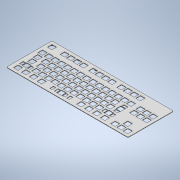
# Autodesk Inventor part: Plate
Saved by Autodesk Inventor 2022 (Build 260153000, 153)
## iProperties
Created: 2021-09-06
Part Number: Plate
Material: 一般
Document SubType Name: Modeling
Designer: shiok
Density: 1 g/cm^3
Appearance: 既定
Author: shiok
## iProperties of the stored document Plate_3D プリント.ipt
Created: 2021-09-06
Part Number: Plate_3D プリント
Material: 一般
Document SubType Name: Modeling
Designer: shiok
Density: 1 g/cm^3
Appearance: 既定
Author: shiok
Autodesk Inventor part; units mm, degrees
(part 1 of 3)
ref_plane "YZ Plane" through (0, 0, 0) normal (1, 0, 0) x (0, 1, 0)
ref_plane "XZ Plane" through (0, 0, 0) normal (0, 1, 0) x (-1, 0, 0)
ref_plane "XY Plane" through (0, 0, 0) normal (0, 0, 1) x (1, 0, 0)
sketch "スケッチ1" plane through (0, 0, 0) normal (0, 1, 0) x (-1, 0, 0)
  line L0 (180.1975, -68.58) -> (-180.1975, -68.58)
  line L1 (-183.1975, -65.58) -> (-183.1975, 65.58)
  line L2 (-180.1975, 68.58) -> (180.1975, 68.58)
  line L3 (183.1975, 65.58) -> (183.1975, -65.58)
  line L4 (183.1975, 68.58) -> (-183.1975, -68.58) construction
  line L5 (183.1975, -68.58) -> (-183.1975, 68.58) construction
  arc A0 (180.1975, -68.58) -> (183.1975, -65.58) centre (180.1975, -65.58) ccw
  arc A1 (183.1975, 65.58) -> (180.1975, 68.58) centre (180.1975, 65.58) ccw
  arc A2 (-180.1975, 68.58) -> (-183.1975, 65.58) centre (-180.1975, 65.58) ccw
  arc A3 (-183.1975, -65.58) -> (-180.1975, -68.58) centre (-180.1975, -65.58) ccw
  line L6 (135.3312, -59.0677) -> (121.8438, -59.0677)
  line L7 (121.5898, -58.8137) -> (121.5898, -45.3263)
  line L8 (121.8438, -45.0723) -> (135.3312, -45.0723)
  line L9 (135.5852, -45.3263) -> (135.5852, -58.8137)
  line L10 (135.5852, -59.0677) -> (121.5898, -45.0723) construction
  line L11 (121.5898, -59.0677) -> (135.5852, -45.0723) construction
  arc A4 (135.3312, -59.0677) -> (135.5852, -58.8137) centre (135.3312, -58.8137) ccw
  arc A5 (121.5898, -58.8137) -> (121.8438, -59.0677) centre (121.8438, -58.8137) ccw
  arc A6 (121.8438, -45.0723) -> (121.5898, -45.3263) centre (121.8438, -45.3263) ccw
  arc A7 (135.5852, -45.3263) -> (135.3312, -45.0723) centre (135.3312, -45.3263) ccw
  line L12 (116.5352, -45.3263) -> (116.5352, -58.8137)
  arc A8 (116.5352, -45.3263) -> (116.2812, -45.0723) centre (116.2812, -45.3263) ccw
  arc A9 (116.2812, -59.0677) -> (116.5352, -58.8137) centre (116.2812, -58.8137) ccw
  line L13 (116.2812, -59.0677) -> (102.7938, -59.0677)
  line L14 (102.7938, -45.0723) -> (116.2812, -45.0723)
  line L15 (116.5352, -59.0677) -> (102.5398, -45.0723) construction
  line L16 (102.5398, -59.0677) -> (116.5352, -45.0723) construction
  arc A10 (102.7938, -45.0723) -> (102.5398, -45.3263) centre (102.7938, -45.3263) ccw
  line L17 (102.5398, -58.8137) -> (102.5398, -45.3263)
  arc A11 (102.5398, -58.8137) -> (102.7938, -59.0677) centre (102.7938, -58.8137) ccw
  line L18 (97.4852, -45.3263) -> (97.4852, -58.8137)
  arc A12 (97.4852, -45.3263) -> (97.2312, -45.0723) centre (97.2312, -45.3263) ccw
  arc A13 (97.2312, -59.0677) -> (97.4852, -58.8137) centre (97.2312, -58.8137) ccw
  line L19 (97.2312, -59.0677) -> (83.7438, -59.0677)
  line L20 (83.7438, -45.0723) -> (97.2312, -45.0723)
  line L21 (97.4852, -59.0677) -> (83.4898, -45.0723) construction
  line L22 (83.4898, -59.0677) -> (97.4852, -45.0723) construction
  arc A14 (83.7438, -45.0723) -> (83.4898, -45.3263) centre (83.7438, -45.3263) ccw
  line L23 (83.4898, -58.8137) -> (83.4898, -45.3263)
  arc A15 (83.4898, -58.8137) -> (83.7438, -59.0677) centre (83.7438, -58.8137) ccw
  line L24 (78.4352, -45.3263) -> (78.4352, -58.8137)
  arc A16 (78.4352, -45.3263) -> (78.1812, -45.0723) centre (78.1812, -45.3263) ccw
  arc A17 (78.1812, -59.0677) -> (78.4352, -58.8137) centre (78.1812, -58.8137) ccw
  line L25 (78.1812, -59.0677) -> (64.6938, -59.0677)
  line L26 (64.6938, -45.0723) -> (78.1812, -45.0723)
  line L27 (78.4352, -59.0677) -> (64.4398, -45.0723) construction
  line L28 (64.4398, -59.0677) -> (78.4352, -45.0723) construction
  arc A18 (64.6938, -45.0723) -> (64.4398, -45.3263) centre (64.6938, -45.3263) ccw
  line L29 (64.4398, -58.8137) -> (64.4398, -45.3263)
  arc A19 (64.4398, -58.8137) -> (64.6938, -59.0677) centre (64.6938, -58.8137) ccw
  line L30 (36.1188, -45.0723) -> (49.6062, -45.0723)
  line L31 (35.8648, -58.8137) -> (35.8648, -45.3263)
  line L32 (49.8602, -45.3263) -> (49.8602, -58.8137)
  line L33 (49.8602, -59.0677) -> (35.8648, -45.0723) construction
  line L34 (35.8648, -59.0677) -> (49.8602, -45.0723) construction
  arc A20 (49.6062, -59.0677) -> (49.8602, -58.8137) centre (49.6062, -58.8137) ccw
  arc A21 (35.8648, -58.8137) -> (36.1188, -59.0677) centre (36.1188, -58.8137) ccw
  line L35 (30.8102, -45.3263) -> (30.8102, -58.8137)
  line L36 (49.6062, -59.0677) -> (36.1188, -59.0677)
  arc A22 (49.8602, -45.3263) -> (49.6062, -45.0723) centre (49.6062, -45.3263) ccw
  arc A23 (36.1188, -45.0723) -> (35.8648, -45.3263) centre (36.1188, -45.3263) ccw
  arc A24 (30.8102, -45.3263) -> (30.5562, -45.0723) centre (30.5562, -45.3263) ccw
  arc A25 (30.5562, -59.0677) -> (30.8102, -58.8137) centre (30.5562, -58.8137) ccw
  line L37 (17.0688, -45.0723) -> (30.5562, -45.0723)
  line L38 (30.5562, -59.0677) -> (17.0688, -59.0677)
  line L39 (30.8102, -59.0677) -> (16.8148, -45.0723) construction
  line L40 (16.8148, -59.0677) -> (30.8102, -45.0723) construction
  arc A26 (17.0688, -45.0723) -> (16.8148, -45.3263) centre (17.0688, -45.3263) ccw
  line L41 (16.8148, -58.8137) -> (16.8148, -45.3263)
  arc A27 (16.8148, -58.8137) -> (17.0688, -59.0677) centre (17.0688, -58.8137) ccw
  line L42 (11.7602, -45.3263) -> (11.7602, -58.8137)
  arc A28 (11.7602, -45.3263) -> (11.5062, -45.0723) centre (11.5062, -45.3263) ccw
  arc A29 (11.5062, -59.0677) -> (11.7602, -58.8137) centre (11.5062, -58.8137) ccw
  line L43 (11.5062, -59.0677) -> (-1.9812, -59.0677)
  line L44 (-1.9812, -45.0723) -> (11.5062, -45.0723)
  line L45 (11.7602, -59.0677) -> (-2.2352, -45.0723) construction
  line L46 (-2.2352, -59.0677) -> (11.7602, -45.0723) construction
  arc A30 (-2.2352, -58.8137) -> (-1.9812, -59.0677) centre (-1.9812, -58.8137) ccw
  arc A31 (-7.5438, -59.0677) -> (-7.2898, -58.8137) centre (-7.5438, -58.8137) ccw
  arc A32 (-1.9812, -45.0723) -> (-2.2352, -45.3263) centre (-1.9812, -45.3263) ccw
  line L47 (-2.2352, -58.8137) -> (-2.2352, -45.3263)
  line L48 (-7.2898, -45.3263) -> (-7.2898, -58.8137)
  line L49 (-7.5438, -59.0677) -> (-21.0312, -59.0677)
  arc A33 (-21.2852, -58.8137) -> (-21.0312, -59.0677) centre (-21.0312, -58.8137) ccw
  arc A34 (-7.2898, -45.3263) -> (-7.5438, -45.0723) centre (-7.5438, -45.3263) ccw
  line L50 (-21.0312, -45.0723) -> (-7.5438, -45.0723)
  line L51 (-21.2852, -58.8137) -> (-21.2852, -45.3263)
  line L52 (-21.2852, -59.0677) -> (-7.2898, -45.0723) construction
  arc A35 (-21.0312, -45.0723) -> (-21.2852, -45.3263) centre (-21.0312, -45.3263) ccw
  line L53 (-7.2898, -59.0677) -> (-21.2852, -45.0723) construction
  line L54 (-49.6062, -45.0723) -> (-36.1188, -45.0723)
  line L55 (-49.8602, -58.8137) -> (-49.8602, -45.3263)
  line L56 (-35.8648, -45.3263) -> (-35.8648, -58.8137)
  line L57 (-35.8648, -59.0677) -> (-49.8602, -45.0723) construction
  line L58 (-49.8602, -59.0677) -> (-35.8648, -45.0723) construction
  arc A36 (-36.1188, -59.0677) -> (-35.8648, -58.8137) centre (-36.1188, -58.8137) ccw
  arc A37 (-49.8602, -58.8137) -> (-49.6062, -59.0677) centre (-49.6062, -58.8137) ccw
  line L59 (-54.9148, -45.3263) -> (-54.9148, -58.8137)
  line L60 (-36.1188, -59.0677) -> (-49.6062, -59.0677)
  arc A38 (-35.8648, -45.3263) -> (-36.1188, -45.0723) centre (-36.1188, -45.3263) ccw
  arc A39 (-49.6062, -45.0723) -> (-49.8602, -45.3263) centre (-49.6062, -45.3263) ccw
  arc A40 (-54.9148, -45.3263) -> (-55.1688, -45.0723) centre (-55.1688, -45.3263) ccw
  arc A41 (-55.1688, -59.0677) -> (-54.9148, -58.8137) centre (-55.1688, -58.8137) ccw
  line L61 (-68.6562, -45.0723) -> (-55.1688, -45.0723)
  line L62 (-55.1688, -59.0677) -> (-68.6562, -59.0677)
  line L63 (-54.9148, -59.0677) -> (-68.9102, -45.0723) construction
  line L64 (-68.9102, -59.0677) -> (-54.9148, -45.0723) construction
  arc A42 (-68.6562, -45.0723) -> (-68.9102, -45.3263) centre (-68.6562, -45.3263) ccw
  line L65 (-68.9102, -58.8137) -> (-68.9102, -45.3263)
  arc A43 (-68.9102, -58.8137) -> (-68.6562, -59.0677) centre (-68.6562, -58.8137) ccw
  line L66 (-73.9648, -45.3263) -> (-73.9648, -58.8137)
  arc A44 (-73.9648, -45.3263) -> (-74.2188, -45.0723) centre (-74.2188, -45.3263) ccw
  arc A45 (-74.2188, -59.0677) -> (-73.9648, -58.8137) centre (-74.2188, -58.8137) ccw
  line L67 (-74.2188, -59.0677) -> (-87.7062, -59.0677)
  line L68 (-87.7062, -45.0723) -> (-74.2188, -45.0723)
  line L69 (-73.9648, -59.0677) -> (-87.9602, -45.0723) construction
  line L70 (-87.9602, -59.0677) -> (-73.9648, -45.0723) construction
  arc A46 (-87.9602, -58.8137) -> (-87.7062, -59.0677) centre (-87.7062, -58.8137) ccw
  arc A47 (-93.2688, -59.0677) -> (-93.0148, -58.8137) centre (-93.2688, -58.8137) ccw
  arc A48 (-87.7062, -45.0723) -> (-87.9602, -45.3263) centre (-87.7062, -45.3263) ccw
  line L71 (-87.9602, -58.8137) -> (-87.9602, -45.3263)
  line L72 (-93.0148, -45.3263) -> (-93.0148, -58.8137)
  line L73 (-93.2688, -59.0677) -> (-106.7562, -59.0677)
  arc A49 (-107.0102, -58.8137) -> (-106.7562, -59.0677) centre (-106.7562, -58.8137) ccw
  arc A50 (-93.0148, -45.3263) -> (-93.2688, -45.0723) centre (-93.2688, -45.3263) ccw
  line L74 (-106.7562, -45.0723) -> (-93.2688, -45.0723)
  line L75 (-107.0102, -58.8137) -> (-107.0102, -45.3263)
  line L76 (-107.0102, -59.0677) -> (-93.0148, -45.0723) construction
  arc A51 (-106.7562, -45.0723) -> (-107.0102, -45.3263) centre (-106.7562, -45.3263) ccw
  line L77 (-93.0148, -59.0677) -> (-107.0102, -45.0723) construction
  line L78 (128.5875, -68.58) -> (128.5875, -52.07) construction
  line L79 (128.5875, -52.07) -> (183.1975, -52.07) construction
  line L80 (173.4312, -30.4927) -> (159.9438, -30.4927)
  line L81 (159.6898, -30.2387) -> (159.6898, -16.7513)
  line L82 (159.9438, -16.4973) -> (173.4312, -16.4973)
  line L83 (173.6852, -16.7513) -> (173.6852, -30.2387)
  line L84 (173.6852, -30.4927) -> (159.6898, -16.4973) construction
  line L85 (159.6898, -30.4927) -> (173.6852, -16.4973) construction
  arc A52 (173.4312, -30.4927) -> (173.6852, -30.2387) centre (173.4312, -30.2387) ccw
  arc A53 (159.6898, -30.2387) -> (159.9438, -30.4927) centre (159.9438, -30.2387) ccw
  arc A54 (159.9438, -16.4973) -> (159.6898, -16.7513) centre (159.9438, -16.7513) ccw
  arc A55 (173.6852, -16.7513) -> (173.4312, -16.4973) centre (173.4312, -16.7513) ccw
  line L86 (76.6706, -116.022) -> (63.1832, -116.022)
  line L87 (62.9292, -115.768) -> (62.9292, -102.2806)
  line L88 (63.1832, -102.0266) -> (76.6706, -102.0266)
  line L89 (76.9246, -102.2806) -> (76.9246, -115.768)
  line L90 (76.9246, -116.022) -> (62.9292, -102.0266) construction
  line L91 (62.9292, -116.022) -> (76.9246, -102.0266) construction
  arc A56 (76.6706, -116.022) -> (76.9246, -115.768) centre (76.6706, -115.768) ccw
  arc A57 (62.9292, -115.768) -> (63.1832, -116.022) centre (63.1832, -115.768) ccw
  arc A58 (63.1832, -102.0266) -> (62.9292, -102.2806) centre (63.1832, -102.2806) ccw
  arc A59 (76.9246, -102.2806) -> (76.6706, -102.0266) centre (76.6706, -102.2806) ccw
  line L92 (173.4312, -59.0677) -> (159.9438, -59.0677)
  line L93 (159.6898, -58.8137) -> (159.6898, -45.3263)
  line L94 (159.9438, -45.0723) -> (173.4312, -45.0723)
  line L95 (173.6852, -45.3263) -> (173.6852, -58.8137)
  line L96 (173.6852, -59.0677) -> (159.6898, -45.0723) construction
  line L97 (159.6898, -59.0677) -> (173.6852, -45.0723) construction
  arc A60 (173.4312, -59.0677) -> (173.6852, -58.8137) centre (173.4312, -58.8137) ccw
  arc A61 (159.6898, -58.8137) -> (159.9438, -59.0677) centre (159.9438, -58.8137) ccw
  arc A62 (159.9438, -45.0723) -> (159.6898, -45.3263) centre (159.9438, -45.3263) ccw
  arc A63 (173.6852, -45.3263) -> (173.4312, -45.0723) centre (173.4312, -45.3263) ccw
  arc A64 (135.5852, 40.3987) -> (135.3312, 40.6527) centre (135.3312, 40.3987) ccw
  line L98 (135.5852, 40.3987) -> (135.5852, 26.9113)
  arc A65 (135.3312, 26.6573) -> (135.5852, 26.9113) centre (135.3312, 26.9113) ccw
  line L99 (121.8438, 40.6527) -> (135.3312, 40.6527)
  line L100 (135.3312, 26.6573) -> (121.8438, 26.6573)
  line L101 (135.5852, 26.6573) -> (121.5898, 40.6527) construction
  line L102 (121.5898, 26.6573) -> (135.5852, 40.6527) construction
  arc A66 (121.5898, 26.9113) -> (121.8438, 26.6573) centre (121.8438, 26.9113) ccw
  line L103 (121.5898, 26.9113) -> (121.5898, 40.3987)
  arc A67 (121.8438, 40.6527) -> (121.5898, 40.3987) centre (121.8438, 40.3987) ccw
  line L104 (154.3812, -30.4927) -> (140.8938, -30.4927)
  line L105 (140.6398, -30.2387) -> (140.6398, -16.7513)
  line L106 (140.8938, -16.4973) -> (154.3812, -16.4973)
  line L107 (154.6352, -16.7513) -> (154.6352, -30.2387)
  line L108 (154.6352, -30.4927) -> (140.6398, -16.4973) construction
  line L109 (140.6398, -30.4927) -> (154.6352, -16.4973) construction
  arc A68 (154.3812, -30.4927) -> (154.6352, -30.2387) centre (154.3812, -30.2387) ccw
  arc A69 (140.6398, -30.2387) -> (140.8938, -30.4927) centre (140.8938, -30.2387) ccw
  arc A70 (140.8938, -16.4973) -> (140.6398, -16.7513) centre (140.8938, -16.7513) ccw
  arc A71 (154.6352, -16.7513) -> (154.3812, -16.4973) centre (154.3812, -16.7513) ccw
  line L110 (135.3312, -30.4927) -> (121.8438, -30.4927)
  line L111 (121.5898, -30.2387) -> (121.5898, -16.7513)
  line L112 (121.8438, -16.4973) -> (135.3312, -16.4973)
  line L113 (135.5852, -16.7513) -> (135.5852, -30.2387)
  line L114 (135.5852, -30.4927) -> (121.5898, -16.4973) construction
  line L115 (121.5898, -30.4927) -> (135.5852, -16.4973) construction
  arc A72 (135.3312, -30.4927) -> (135.5852, -30.2387) centre (135.3312, -30.2387) ccw
  arc A73 (121.5898, -30.2387) -> (121.8438, -30.4927) centre (121.8438, -30.2387) ccw
  arc A74 (121.8438, -16.4973) -> (121.5898, -16.7513) centre (121.8438, -16.7513) ccw
  arc A75 (135.5852, -16.7513) -> (135.3312, -16.4973) centre (135.3312, -16.7513) ccw
  line L116 (116.2812, -30.4927) -> (102.7938, -30.4927)
  line L117 (102.5398, -30.2387) -> (102.5398, -16.7513)
  line L118 (102.7938, -16.4973) -> (116.2812, -16.4973)
  line L119 (116.5352, -16.7513) -> (116.5352, -30.2387)
  line L120 (116.5352, -30.4927) -> (102.5398, -16.4973) construction
  line L121 (102.5398, -30.4927) -> (116.5352, -16.4973) construction
  arc A76 (116.2812, -30.4927) -> (116.5352, -30.2387) centre (116.2812, -30.2387) ccw
  arc A77 (102.5398, -30.2387) -> (102.7938, -30.4927) centre (102.7938, -30.2387) ccw
  arc A78 (102.7938, -16.4973) -> (102.5398, -16.7513) centre (102.7938, -16.7513) ccw
  arc A79 (116.5352, -16.7513) -> (116.2812, -16.4973) centre (116.2812, -16.7513) ccw
  line L122 (97.2312, -30.4927) -> (83.7438, -30.4927)
  line L123 (83.4898, -30.2387) -> (83.4898, -16.7513)
  line L124 (83.7438, -16.4973) -> (97.2312, -16.4973)
  line L125 (97.4852, -16.7513) -> (97.4852, -30.2387)
  line L126 (97.4852, -30.4927) -> (83.4898, -16.4973) construction
  line L127 (83.4898, -30.4927) -> (97.4852, -16.4973) construction
  arc A80 (97.2312, -30.4927) -> (97.4852, -30.2387) centre (97.2312, -30.2387) ccw
  arc A81 (83.4898, -30.2387) -> (83.7438, -30.4927) centre (83.7438, -30.2387) ccw
  arc A82 (83.7438, -16.4973) -> (83.4898, -16.7513) centre (83.7438, -16.7513) ccw
  arc A83 (97.4852, -16.7513) -> (97.2312, -16.4973) centre (97.2312, -16.7513) ccw
  line L128 (78.1812, -30.4927) -> (64.6938, -30.4927)
  line L129 (64.4398, -30.2387) -> (64.4398, -16.7513)
  line L130 (64.6938, -16.4973) -> (78.1812, -16.4973)
  line L131 (78.4352, -16.7513) -> (78.4352, -30.2387)
  line L132 (78.4352, -30.4927) -> (64.4398, -16.4973) construction
  line L133 (64.4398, -30.4927) -> (78.4352, -16.4973) construction
  arc A84 (78.1812, -30.4927) -> (78.4352, -30.2387) centre (78.1812, -30.2387) ccw
  arc A85 (64.4398, -30.2387) -> (64.6938, -30.4927) centre (64.6938, -30.2387) ccw
  arc A86 (64.6938, -16.4973) -> (64.4398, -16.7513) centre (64.6938, -16.7513) ccw
  arc A87 (78.4352, -16.7513) -> (78.1812, -16.4973) centre (78.1812, -16.7513) ccw
  line L134 (59.1312, -30.4927) -> (45.6438, -30.4927)
  line L135 (45.3898, -30.2387) -> (45.3898, -16.7513)
  line L136 (45.6438, -16.4973) -> (59.1312, -16.4973)
  line L137 (59.3852, -16.7513) -> (59.3852, -30.2387)
  line L138 (59.3852, -30.4927) -> (45.3898, -16.4973) construction
  line L139 (45.3898, -30.4927) -> (59.3852, -16.4973) construction
  arc A88 (59.1312, -30.4927) -> (59.3852, -30.2387) centre (59.1312, -30.2387) ccw
  arc A89 (45.3898, -30.2387) -> (45.6438, -30.4927) centre (45.6438, -30.2387) ccw
  arc A90 (45.6438, -16.4973) -> (45.3898, -16.7513) centre (45.6438, -16.7513) ccw
  arc A91 (59.3852, -16.7513) -> (59.1312, -16.4973) centre (59.1312, -16.7513) ccw
  line L140 (40.0812, -30.4927) -> (26.5938, -30.4927)
  line L141 (26.3398, -30.2387) -> (26.3398, -16.7513)
  line L142 (26.5938, -16.4973) -> (40.0812, -16.4973)
  line L143 (40.3352, -16.7513) -> (40.3352, -30.2387)
  line L144 (40.3352, -30.4927) -> (26.3398, -16.4973) construction
  line L145 (26.3398, -30.4927) -> (40.3352, -16.4973) construction
  arc A92 (40.0812, -30.4927) -> (40.3352, -30.2387) centre (40.0812, -30.2387) ccw
  arc A93 (26.3398, -30.2387) -> (26.5938, -30.4927) centre (26.5938, -30.2387) ccw
  arc A94 (26.5938, -16.4973) -> (26.3398, -16.7513) centre (26.5938, -16.7513) ccw
  arc A95 (40.3352, -16.7513) -> (40.0812, -16.4973) centre (40.0812, -16.7513) ccw
  line L146 (21.0312, -30.4927) -> (7.5438, -30.4927)
  line L147 (7.2898, -30.2387) -> (7.2898, -16.7513)
  line L148 (7.5438, -16.4973) -> (21.0312, -16.4973)
  line L149 (21.2852, -16.7513) -> (21.2852, -30.2387)
  line L150 (21.2852, -30.4927) -> (7.2898, -16.4973) construction
  line L151 (7.2898, -30.4927) -> (21.2852, -16.4973) construction
  arc A96 (21.0312, -30.4927) -> (21.2852, -30.2387) centre (21.0312, -30.2387) ccw
  arc A97 (7.2898, -30.2387) -> (7.5438, -30.4927) centre (7.5438, -30.2387) ccw
  arc A98 (7.5438, -16.4973) -> (7.2898, -16.7513) centre (7.5438, -16.7513) ccw
  arc A99 (21.2852, -16.7513) -> (21.0312, -16.4973) centre (21.0312, -16.7513) ccw
  line L152 (1.9812, -30.4927) -> (-11.5062, -30.4927)
  line L153 (-11.7602, -30.2387) -> (-11.7602, -16.7513)
  line L154 (-11.5062, -16.4973) -> (1.9812, -16.4973)
  line L155 (2.2352, -16.7513) -> (2.2352, -30.2387)
  line L156 (2.2352, -30.4927) -> (-11.7602, -16.4973) construction
  line L157 (-11.7602, -30.4927) -> (2.2352, -16.4973) construction
  arc A100 (1.9812, -30.4927) -> (2.2352, -30.2387) centre (1.9812, -30.2387) ccw
  arc A101 (-11.7602, -30.2387) -> (-11.5062, -30.4927) centre (-11.5062, -30.2387) ccw
  arc A102 (-11.5062, -16.4973) -> (-11.7602, -16.7513) centre (-11.5062, -16.7513) ccw
  arc A103 (2.2352, -16.7513) -> (1.9812, -16.4973) centre (1.9812, -16.7513) ccw
  line L158 (-17.0688, -30.4927) -> (-30.5562, -30.4927)
  line L159 (-30.8102, -30.2387) -> (-30.8102, -16.7513)
  line L160 (-30.5562, -16.4973) -> (-17.0688, -16.4973)
  line L161 (-16.8148, -16.7513) -> (-16.8148, -30.2387)
  line L162 (-16.8148, -30.4927) -> (-30.8102, -16.4973) construction
  line L163 (-30.8102, -30.4927) -> (-16.8148, -16.4973) construction
  arc A104 (-17.0688, -30.4927) -> (-16.8148, -30.2387) centre (-17.0688, -30.2387) ccw
  arc A105 (-30.8102, -30.2387) -> (-30.5562, -30.4927) centre (-30.5562, -30.2387) ccw
  arc A106 (-30.5562, -16.4973) -> (-30.8102, -16.7513) centre (-30.5562, -16.7513) ccw
  arc A107 (-16.8148, -16.7513) -> (-17.0688, -16.4973) centre (-17.0688, -16.7513) ccw
  line L164 (-36.1188, -30.4927) -> (-49.6062, -30.4927)
  line L165 (-49.8602, -30.2387) -> (-49.8602, -16.7513)
  line L166 (-49.6062, -16.4973) -> (-36.1188, -16.4973)
  line L167 (-35.8648, -16.7513) -> (-35.8648, -30.2387)
  line L168 (-35.8648, -30.4927) -> (-49.8602, -16.4973) construction
  line L169 (-49.8602, -30.4927) -> (-35.8648, -16.4973) construction
  arc A108 (-36.1188, -30.4927) -> (-35.8648, -30.2387) centre (-36.1188, -30.2387) ccw
  arc A109 (-49.8602, -30.2387) -> (-49.6062, -30.4927) centre (-49.6062, -30.2387) ccw
  arc A110 (-49.6062, -16.4973) -> (-49.8602, -16.7513) centre (-49.6062, -16.7513) ccw
  arc A111 (-35.8648, -16.7513) -> (-36.1188, -16.4973) centre (-36.1188, -16.7513) ccw
  line L170 (-55.1688, -30.4927) -> (-68.6562, -30.4927)
  line L171 (-68.9102, -30.2387) -> (-68.9102, -16.7513)
  line L172 (-68.6562, -16.4973) -> (-55.1688, -16.4973)
  line L173 (-54.9148, -16.7513) -> (-54.9148, -30.2387)
  line L174 (-54.9148, -30.4927) -> (-68.9102, -16.4973) construction
  line L175 (-68.9102, -30.4927) -> (-54.9148, -16.4973) construction
  arc A112 (-55.1688, -30.4927) -> (-54.9148, -30.2387) centre (-55.1688, -30.2387) ccw
  arc A113 (-68.9102, -30.2387) -> (-68.6562, -30.4927) centre (-68.6562, -30.2387) ccw
  arc A114 (-68.6562, -16.4973) -> (-68.9102, -16.7513) centre (-68.6562, -16.7513) ccw
  arc A115 (-54.9148, -16.7513) -> (-55.1688, -16.4973) centre (-55.1688, -16.7513) ccw
  line L176 (-74.2188, -30.4927) -> (-87.7062, -30.4927)
  line L177 (-87.9602, -30.2387) -> (-87.9602, -16.7513)
  line L178 (-87.7062, -16.4973) -> (-74.2188, -16.4973)
  line L179 (-73.9648, -16.7513) -> (-73.9648, -30.2387)
  line L180 (-73.9648, -30.4927) -> (-87.9602, -16.4973) construction
  line L181 (-87.9602, -30.4927) -> (-73.9648, -16.4973) construction
  arc A116 (-74.2188, -30.4927) -> (-73.9648, -30.2387) centre (-74.2188, -30.2387) ccw
  arc A117 (-87.9602, -30.2387) -> (-87.7062, -30.4927) centre (-87.7062, -30.2387) ccw
  arc A118 (-87.7062, -16.4973) -> (-87.9602, -16.7513) centre (-87.7062, -16.7513) ccw
  arc A119 (-73.9648, -16.7513) -> (-74.2188, -16.4973) centre (-74.2188, -16.7513) ccw
  line L182 (-93.2688, -30.4927) -> (-106.7562, -30.4927)
  line L183 (-107.0102, -30.2387) -> (-107.0102, -16.7513)
  line L184 (-106.7562, -16.4973) -> (-93.2688, -16.4973)
  line L185 (-93.0148, -16.7513) -> (-93.0148, -30.2387)
  line L186 (-93.0148, -30.4927) -> (-107.0102, -16.4973) construction
  line L187 (-107.0102, -30.4927) -> (-93.0148, -16.4973) construction
  arc A120 (-93.2688, -30.4927) -> (-93.0148, -30.2387) centre (-93.2688, -30.2387) ccw
  arc A121 (-107.0102, -30.2387) -> (-106.7562, -30.4927) centre (-106.7562, -30.2387) ccw
  arc A122 (-106.7562, -16.4973) -> (-107.0102, -16.7513) centre (-106.7562, -16.7513) ccw
  arc A123 (-93.0148, -16.7513) -> (-93.2688, -16.4973) centre (-93.2688, -16.7513) ccw
  line L188 (166.6875, -68.58) -> (166.6875, 68.58) construction
  arc A124 (131.3688, 2.5527) -> (131.1148, 2.2987) centre (131.3688, 2.2987) ccw
  line L189 (131.1148, -11.1887) -> (131.1148, 2.2987)
  arc A125 (131.1148, -11.1887) -> (131.3688, -11.4427) centre (131.3688, -11.1887) ccw
  line L190 (131.3688, 2.5527) -> (144.8562, 2.5527)
  arc A126 (145.1102, 2.2987) -> (144.8562, 2.5527) centre (144.8562, 2.2987) ccw
  line L191 (144.8562, -11.4427) -> (131.3688, -11.4427)
  line L192 (145.1102, -11.4427) -> (131.1148, 2.5527) construction
  line L193 (131.1148, -11.4427) -> (145.1102, 2.5527) construction
  line L194 (145.1102, 2.2987) -> (145.1102, -11.1887)
  arc A127 (144.8562, -11.4427) -> (145.1102, -11.1887) centre (144.8562, -11.1887) ccw
  arc A128 (112.3188, 2.5527) -> (112.0648, 2.2987) centre (112.3188, 2.2987) ccw
  line L195 (112.3188, 2.5527) -> (125.8062, 2.5527)
  line L196 (112.0648, -11.1887) -> (112.0648, 2.2987)
  arc A129 (112.0648, -11.1887) -> (112.3188, -11.4427) centre (112.3188, -11.1887) ccw
  line L197 (125.8062, -11.4427) -> (112.3188, -11.4427)
  line L198 (112.0648, -11.4427) -> (126.0602, 2.5527) construction
  line L199 (126.0602, -11.4427) -> (112.0648, 2.5527) construction
  line L200 (126.0602, 2.2987) -> (126.0602, -11.1887)
  arc A130 (125.8062, -11.4427) -> (126.0602, -11.1887) centre (125.8062, -11.1887) ccw
  arc A131 (126.0602, 2.2987) -> (125.8062, 2.5527) centre (125.8062, 2.2987) ccw
  arc A132 (93.2688, 2.5527) -> (93.0148, 2.2987) centre (93.2688, 2.2987) ccw
  line L201 (93.2688, 2.5527) -> (106.7562, 2.5527)
  line L202 (93.0148, -11.1887) -> (93.0148, 2.2987)
  arc A133 (93.0148, -11.1887) -> (93.2688, -11.4427) centre (93.2688, -11.1887) ccw
  line L203 (106.7562, -11.4427) -> (93.2688, -11.4427)
  line L204 (93.0148, -11.4427) -> (107.0102, 2.5527) construction
  line L205 (107.0102, -11.4427) -> (93.0148, 2.5527) construction
  line L206 (107.0102, 2.2987) -> (107.0102, -11.1887)
  arc A134 (106.7562, -11.4427) -> (107.0102, -11.1887) centre (106.7562, -11.1887) ccw
  arc A135 (107.0102, 2.2987) -> (106.7562, 2.5527) centre (106.7562, 2.2987) ccw
  arc A136 (74.2188, 2.5527) -> (73.9648, 2.2987) centre (74.2188, 2.2987) ccw
  line L207 (74.2188, 2.5527) -> (87.7062, 2.5527)
  line L208 (73.9648, -11.1887) -> (73.9648, 2.2987)
  arc A137 (73.9648, -11.1887) -> (74.2188, -11.4427) centre (74.2188, -11.1887) ccw
  line L209 (87.7062, -11.4427) -> (74.2188, -11.4427)
  line L210 (73.9648, -11.4427) -> (87.9602, 2.5527) construction
  line L211 (87.9602, -11.4427) -> (73.9648, 2.5527) construction
  line L212 (87.9602, 2.2987) -> (87.9602, -11.1887)
  arc A138 (87.7062, -11.4427) -> (87.9602, -11.1887) centre (87.7062, -11.1887) ccw
  arc A139 (87.9602, 2.2987) -> (87.7062, 2.5527) centre (87.7062, 2.2987) ccw
  arc A140 (55.1688, 2.5527) -> (54.9148, 2.2987) centre (55.1688, 2.2987) ccw
  line L213 (55.1688, 2.5527) -> (68.6562, 2.5527)
  line L214 (54.9148, -11.1887) -> (54.9148, 2.2987)
  arc A141 (54.9148, -11.1887) -> (55.1688, -11.4427) centre (55.1688, -11.1887) ccw
  line L215 (68.6562, -11.4427) -> (55.1688, -11.4427)
  line L216 (54.9148, -11.4427) -> (68.9102, 2.5527) construction
  line L217 (68.9102, -11.4427) -> (54.9148, 2.5527) construction
  line L218 (68.9102, 2.2987) -> (68.9102, -11.1887)
  arc A142 (68.6562, -11.4427) -> (68.9102, -11.1887) centre (68.6562, -11.1887) ccw
  arc A143 (68.9102, 2.2987) -> (68.6562, 2.5527) centre (68.6562, 2.2987) ccw
  arc A144 (36.1188, 2.5527) -> (35.8648, 2.2987) centre (36.1188, 2.2987) ccw
  line L219 (36.1188, 2.5527) -> (49.6062, 2.5527)
  line L220 (35.8648, -11.1887) -> (35.8648, 2.2987)
  arc A145 (35.8648, -11.1887) -> (36.1188, -11.4427) centre (36.1188, -11.1887) ccw
  line L221 (49.6062, -11.4427) -> (36.1188, -11.4427)
  line L222 (35.8648, -11.4427) -> (49.8602, 2.5527) construction
  line L223 (49.8602, -11.4427) -> (35.8648, 2.5527) construction
  line L224 (49.8602, 2.2987) -> (49.8602, -11.1887)
  arc A146 (49.6062, -11.4427) -> (49.8602, -11.1887) centre (49.6062, -11.1887) ccw
  arc A147 (49.8602, 2.2987) -> (49.6062, 2.5527) centre (49.6062, 2.2987) ccw
  arc A148 (17.0688, 2.5527) -> (16.8148, 2.2987) centre (17.0688, 2.2987) ccw
  line L225 (17.0688, 2.5527) -> (30.5562, 2.5527)
  line L226 (16.8148, -11.1887) -> (16.8148, 2.2987)
  arc A149 (16.8148, -11.1887) -> (17.0688, -11.4427) centre (17.0688, -11.1887) ccw
  line L227 (30.5562, -11.4427) -> (17.0688, -11.4427)
  line L228 (16.8148, -11.4427) -> (30.8102, 2.5527) construction
  line L229 (30.8102, -11.4427) -> (16.8148, 2.5527) construction
  line L230 (30.8102, 2.2987) -> (30.8102, -11.1887)
  arc A150 (30.5562, -11.4427) -> (30.8102, -11.1887) centre (30.5562, -11.1887) ccw
  arc A151 (30.8102, 2.2987) -> (30.5562, 2.5527) centre (30.5562, 2.2987) ccw
  arc A152 (-1.9812, 2.5527) -> (-2.2352, 2.2987) centre (-1.9812, 2.2987) ccw
  line L231 (-1.9812, 2.5527) -> (11.5062, 2.5527)
  line L232 (-2.2352, -11.1887) -> (-2.2352, 2.2987)
  arc A153 (-2.2352, -11.1887) -> (-1.9812, -11.4427) centre (-1.9812, -11.1887) ccw
  line L233 (11.5062, -11.4427) -> (-1.9812, -11.4427)
  line L234 (-2.2352, -11.4427) -> (11.7602, 2.5527) construction
  line L235 (11.7602, -11.4427) -> (-2.2352, 2.5527) construction
  line L236 (11.7602, 2.2987) -> (11.7602, -11.1887)
  arc A154 (11.5062, -11.4427) -> (11.7602, -11.1887) centre (11.5062, -11.1887) ccw
  arc A155 (11.7602, 2.2987) -> (11.5062, 2.5527) centre (11.5062, 2.2987) ccw
  arc A156 (-21.0312, 2.5527) -> (-21.2852, 2.2987) centre (-21.0312, 2.2987) ccw
  line L237 (-21.0312, 2.5527) -> (-7.5438, 2.5527)
  line L238 (-21.2852, -11.1887) -> (-21.2852, 2.2987)
  arc A157 (-21.2852, -11.1887) -> (-21.0312, -11.4427) centre (-21.0312, -11.1887) ccw
  line L239 (-7.5438, -11.4427) -> (-21.0312, -11.4427)
  line L240 (-21.2852, -11.4427) -> (-7.2898, 2.5527) construction
  line L241 (-7.2898, -11.4427) -> (-21.2852, 2.5527) construction
  line L242 (-7.2898, 2.2987) -> (-7.2898, -11.1887)
  arc A158 (-7.5438, -11.4427) -> (-7.2898, -11.1887) centre (-7.5438, -11.1887) ccw
  arc A159 (-7.2898, 2.2987) -> (-7.5438, 2.5527) centre (-7.5438, 2.2987) ccw
  arc A160 (-40.0812, 2.5527) -> (-40.3352, 2.2987) centre (-40.0812, 2.2987) ccw
  line L243 (-40.0812, 2.5527) -> (-26.5938, 2.5527)
  line L244 (-40.3352, -11.1887) -> (-40.3352, 2.2987)
  arc A161 (-40.3352, -11.1887) -> (-40.0812, -11.4427) centre (-40.0812, -11.1887) ccw
  line L245 (-26.5938, -11.4427) -> (-40.0812, -11.4427)
  line L246 (-40.3352, -11.4427) -> (-26.3398, 2.5527) construction
  line L247 (-26.3398, -11.4427) -> (-40.3352, 2.5527) construction
  line L248 (-26.3398, 2.2987) -> (-26.3398, -11.1887)
  arc A162 (-26.5938, -11.4427) -> (-26.3398, -11.1887) centre (-26.5938, -11.1887) ccw
  arc A163 (-26.3398, 2.2987) -> (-26.5938, 2.5527) centre (-26.5938, 2.2987) ccw
  arc A164 (-59.1312, 2.5527) -> (-59.3852, 2.2987) centre (-59.1312, 2.2987) ccw
  line L249 (-59.1312, 2.5527) -> (-45.6438, 2.5527)
  line L250 (-59.3852, -11.1887) -> (-59.3852, 2.2987)
  arc A165 (-59.3852, -11.1887) -> (-59.1312, -11.4427) centre (-59.1312, -11.1887) ccw
  line L251 (-45.6438, -11.4427) -> (-59.1312, -11.4427)
  line L252 (-59.3852, -11.4427) -> (-45.3898, 2.5527) construction
  line L253 (-45.3898, -11.4427) -> (-59.3852, 2.5527) construction
  line L254 (-45.3898, 2.2987) -> (-45.3898, -11.1887)
  arc A166 (-45.6438, -11.4427) -> (-45.3898, -11.1887) centre (-45.6438, -11.1887) ccw
  arc A167 (-45.3898, 2.2987) -> (-45.6438, 2.5527) centre (-45.6438, 2.2987) ccw
  arc A168 (-78.1812, 2.5527) -> (-78.4352, 2.2987) centre (-78.1812, 2.2987) ccw
  line L255 (-78.1812, 2.5527) -> (-64.6938, 2.5527)
  line L256 (-78.4352, -11.1887) -> (-78.4352, 2.2987)
  arc A169 (-78.4352, -11.1887) -> (-78.1812, -11.4427) centre (-78.1812, -11.1887) ccw
  line L257 (-64.6938, -11.4427) -> (-78.1812, -11.4427)
  line L258 (-78.4352, -11.4427) -> (-64.4398, 2.5527) construction
  line L259 (-64.4398, -11.4427) -> (-78.4352, 2.5527) construction
  line L260 (-64.4398, 2.2987) -> (-64.4398, -11.1887)
  arc A170 (-64.6938, -11.4427) -> (-64.4398, -11.1887) centre (-64.6938, -11.1887) ccw
  arc A171 (-64.4398, 2.2987) -> (-64.6938, 2.5527) centre (-64.6938, 2.2987) ccw
  line L261 (183.1975, -4.445) -> (138.1125, -4.445) construction
  arc A172 (126.6063, 21.6027) -> (126.3523, 21.3487) centre (126.6063, 21.3487) ccw
  line L262 (126.3523, 7.8613) -> (126.3523, 21.3487)
  arc A173 (126.3523, 7.8613) -> (126.6063, 7.6073) centre (126.6063, 7.8613) ccw
  line L263 (126.6063, 21.6027) -> (140.0937, 21.6027)
  arc A174 (140.3477, 21.3487) -> (140.0937, 21.6027) centre (140.0937, 21.3487) ccw
  line L264 (140.0937, 7.6073) -> (126.6063, 7.6073)
  line L265 (140.3477, 7.6073) -> (126.3523, 21.6027) construction
  line L266 (126.3523, 7.6073) -> (140.3477, 21.6027) construction
  line L267 (140.3477, 21.3487) -> (140.3477, 7.8613)
  arc A175 (140.0937, 7.6073) -> (140.3477, 7.8613) centre (140.0937, 7.8613) ccw
  arc A176 (121.2977, 21.3487) -> (121.0437, 21.6027) centre (121.0437, 21.3487) ccw
  line L268 (121.2977, 21.3487) -> (121.2977, 7.8613)
  arc A177 (121.0437, 7.6073) -> (121.2977, 7.8613) centre (121.0437, 7.8613) ccw
  line L269 (121.0437, 7.6073) -> (107.5563, 7.6073)
  line L270 (107.5563, 21.6027) -> (121.0437, 21.6027)
  line L271 (121.2977, 7.6073) -> (107.3023, 21.6027) construction
  line L272 (107.3023, 7.6073) -> (121.2977, 21.6027) construction
  arc A178 (107.3023, 7.8613) -> (107.5563, 7.6073) centre (107.5563, 7.8613) ccw
  line L273 (107.3023, 7.8613) -> (107.3023, 21.3487)
  arc A179 (107.5563, 21.6027) -> (107.3023, 21.3487) centre (107.5563, 21.3487) ccw
  arc A180 (102.2477, 21.3487) -> (101.9937, 21.6027) centre (101.9937, 21.3487) ccw
  line L274 (102.2477, 21.3487) -> (102.2477, 7.8613)
  arc A181 (101.9937, 7.6073) -> (102.2477, 7.8613) centre (101.9937, 7.8613) ccw
  line L275 (101.9937, 7.6073) -> (88.5063, 7.6073)
  line L276 (88.5063, 21.6027) -> (101.9937, 21.6027)
  line L277 (102.2477, 7.6073) -> (88.2523, 21.6027) construction
  line L278 (88.2523, 7.6073) -> (102.2477, 21.6027) construction
  arc A182 (88.2523, 7.8613) -> (88.5063, 7.6073) centre (88.5063, 7.8613) ccw
  line L279 (88.2523, 7.8613) -> (88.2523, 21.3487)
  arc A183 (88.5063, 21.6027) -> (88.2523, 21.3487) centre (88.5063, 21.3487) ccw
  arc A184 (83.1977, 21.3487) -> (82.9437, 21.6027) centre (82.9437, 21.3487) ccw
  line L280 (83.1977, 21.3487) -> (83.1977, 7.8613)
  arc A185 (82.9437, 7.6073) -> (83.1977, 7.8613) centre (82.9437, 7.8613) ccw
  line L281 (82.9437, 7.6073) -> (69.4563, 7.6073)
  line L282 (69.4563, 21.6027) -> (82.9437, 21.6027)
  line L283 (83.1977, 7.6073) -> (69.2023, 21.6027) construction
  line L284 (69.2023, 7.6073) -> (83.1977, 21.6027) construction
  arc A186 (69.2023, 7.8613) -> (69.4563, 7.6073) centre (69.4563, 7.8613) ccw
  line L285 (69.2023, 7.8613) -> (69.2023, 21.3487)
  arc A187 (69.4563, 21.6027) -> (69.2023, 21.3487) centre (69.4563, 21.3487) ccw
  arc A188 (64.1477, 21.3487) -> (63.8937, 21.6027) centre (63.8937, 21.3487) ccw
  line L286 (64.1477, 21.3487) -> (64.1477, 7.8613)
  arc A189 (63.8937, 7.6073) -> (64.1477, 7.8613) centre (63.8937, 7.8613) ccw
  line L287 (63.8937, 7.6073) -> (50.4063, 7.6073)
  line L288 (50.4063, 21.6027) -> (63.8937, 21.6027)
  line L289 (64.1477, 7.6073) -> (50.1523, 21.6027) construction
  line L290 (50.1523, 7.6073) -> (64.1477, 21.6027) construction
  arc A190 (50.1523, 7.8613) -> (50.4063, 7.6073) centre (50.4063, 7.8613) ccw
  line L291 (50.1523, 7.8613) -> (50.1523, 21.3487)
  arc A191 (50.4063, 21.6027) -> (50.1523, 21.3487) centre (50.4063, 21.3487) ccw
  arc A192 (45.0977, 21.3487) -> (44.8437, 21.6027) centre (44.8437, 21.3487) ccw
  line L292 (45.0977, 21.3487) -> (45.0977, 7.8613)
  arc A193 (44.8437, 7.6073) -> (45.0977, 7.8613) centre (44.8437, 7.8613) ccw
  line L293 (44.8437, 7.6073) -> (31.3563, 7.6073)
  line L294 (31.3563, 21.6027) -> (44.8437, 21.6027)
  line L295 (45.0977, 7.6073) -> (31.1023, 21.6027) construction
  line L296 (31.1023, 7.6073) -> (45.0977, 21.6027) construction
  arc A194 (31.1023, 7.8613) -> (31.3563, 7.6073) centre (31.3563, 7.8613) ccw
  line L297 (31.1023, 7.8613) -> (31.1023, 21.3487)
  arc A195 (31.3563, 21.6027) -> (31.1023, 21.3487) centre (31.3563, 21.3487) ccw
  arc A196 (26.0477, 21.3487) -> (25.7937, 21.6027) centre (25.7937, 21.3487) ccw
  line L298 (26.0477, 21.3487) -> (26.0477, 7.8613)
  arc A197 (25.7937, 7.6073) -> (26.0477, 7.8613) centre (25.7937, 7.8613) ccw
  line L299 (25.7937, 7.6073) -> (12.3063, 7.6073)
  line L300 (12.3063, 21.6027) -> (25.7937, 21.6027)
  line L301 (26.0477, 7.6073) -> (12.0523, 21.6027) construction
  line L302 (12.0523, 7.6073) -> (26.0477, 21.6027) construction
  arc A198 (12.0523, 7.8613) -> (12.3063, 7.6073) centre (12.3063, 7.8613) ccw
  line L303 (12.0523, 7.8613) -> (12.0523, 21.3487)
  arc A199 (12.3063, 21.6027) -> (12.0523, 21.3487) centre (12.3063, 21.3487) ccw
  arc A200 (6.9977, 21.3487) -> (6.7437, 21.6027) centre (6.7437, 21.3487) ccw
  line L304 (6.9977, 21.3487) -> (6.9977, 7.8613)
  arc A201 (6.7437, 7.6073) -> (6.9977, 7.8613) centre (6.7437, 7.8613) ccw
  line L305 (6.7437, 7.6073) -> (-6.7437, 7.6073)
  line L306 (-6.7437, 21.6027) -> (6.7437, 21.6027)
  line L307 (6.9977, 7.6073) -> (-6.9977, 21.6027) construction
  line L308 (-6.9977, 7.6073) -> (6.9977, 21.6027) construction
  arc A202 (-6.9977, 7.8613) -> (-6.7437, 7.6073) centre (-6.7437, 7.8613) ccw
  line L309 (-6.9977, 7.8613) -> (-6.9977, 21.3487)
  arc A203 (-6.7437, 21.6027) -> (-6.9977, 21.3487) centre (-6.7437, 21.3487) ccw
  arc A204 (-12.0523, 21.3487) -> (-12.3063, 21.6027) centre (-12.3063, 21.3487) ccw
  line L310 (-12.0523, 21.3487) -> (-12.0523, 7.8613)
  arc A205 (-12.3063, 7.6073) -> (-12.0523, 7.8613) centre (-12.3063, 7.8613) ccw
  line L311 (-12.3063, 7.6073) -> (-25.7937, 7.6073)
  line L312 (-25.7937, 21.6027) -> (-12.3063, 21.6027)
  line L313 (-12.0523, 7.6073) -> (-26.0477, 21.6027) construction
  line L314 (-26.0477, 7.6073) -> (-12.0523, 21.6027) construction
  arc A206 (-26.0477, 7.8613) -> (-25.7937, 7.6073) centre (-25.7937, 7.8613) ccw
  line L315 (-26.0477, 7.8613) -> (-26.0477, 21.3487)
  arc A207 (-25.7937, 21.6027) -> (-26.0477, 21.3487) centre (-25.7937, 21.3487) ccw
  arc A208 (-31.1023, 21.3487) -> (-31.3563, 21.6027) centre (-31.3563, 21.3487) ccw
  line L316 (-31.1023, 21.3487) -> (-31.1023, 7.8613)
  arc A209 (-31.3563, 7.6073) -> (-31.1023, 7.8613) centre (-31.3563, 7.8613) ccw
  line L317 (-31.3563, 7.6073) -> (-44.8437, 7.6073)
  line L318 (-44.8437, 21.6027) -> (-31.3563, 21.6027)
  line L319 (-31.1023, 7.6073) -> (-45.0977, 21.6027) construction
  line L320 (-45.0977, 7.6073) -> (-31.1023, 21.6027) construction
  arc A210 (-45.0977, 7.8613) -> (-44.8437, 7.6073) centre (-44.8437, 7.8613) ccw
  line L321 (-45.0977, 7.8613) -> (-45.0977, 21.3487)
  arc A211 (-44.8437, 21.6027) -> (-45.0977, 21.3487) centre (-44.8437, 21.3487) ccw
  arc A212 (-50.1523, 21.3487) -> (-50.4063, 21.6027) centre (-50.4063, 21.3487) ccw
  line L322 (-50.1523, 21.3487) -> (-50.1523, 7.8613)
  arc A213 (-50.4063, 7.6073) -> (-50.1523, 7.8613) centre (-50.4063, 7.8613) ccw
  line L323 (-50.4063, 7.6073) -> (-63.8937, 7.6073)
  line L324 (-63.8937, 21.6027) -> (-50.4063, 21.6027)
  line L325 (-50.1523, 7.6073) -> (-64.1477, 21.6027) construction
  line L326 (-64.1477, 7.6073) -> (-50.1523, 21.6027) construction
  arc A214 (-64.1477, 7.8613) -> (-63.8937, 7.6073) centre (-63.8937, 7.8613) ccw
  line L327 (-64.1477, 7.8613) -> (-64.1477, 21.3487)
  arc A215 (-63.8937, 21.6027) -> (-64.1477, 21.3487) centre (-63.8937, 21.3487) ccw
  arc A216 (-69.2023, 21.3487) -> (-69.4563, 21.6027) centre (-69.4563, 21.3487) ccw
  line L328 (-69.2023, 21.3487) -> (-69.2023, 7.8613)
  arc A217 (-69.4563, 7.6073) -> (-69.2023, 7.8613) centre (-69.4563, 7.8613) ccw
  line L329 (-69.4563, 7.6073) -> (-82.9437, 7.6073)
  line L330 (-82.9437, 21.6027) -> (-69.4563, 21.6027)
  line L331 (-69.2023, 7.6073) -> (-83.1977, 21.6027) construction
  line L332 (-83.1977, 7.6073) -> (-69.2023, 21.6027) construction
  arc A218 (-83.1977, 7.8613) -> (-82.9437, 7.6073) centre (-82.9437, 7.8613) ccw
  line L333 (-83.1977, 7.8613) -> (-83.1977, 21.3487)
  arc A219 (-82.9437, 21.6027) -> (-83.1977, 21.3487) centre (-82.9437, 21.3487) ccw
  line L334 (183.1975, 14.605) -> (133.35, 14.605) construction
  arc A220 (152.7988, 21.6027) -> (152.5448, 21.3487) centre (152.7988, 21.3487) ccw
  line L335 (152.5448, 7.8613) -> (152.5448, 21.3487)
  arc A221 (152.5448, 7.8613) -> (152.7988, 7.6073) centre (152.7988, 7.8613) ccw
  line L336 (152.7988, 21.6027) -> (166.2862, 21.6027)
  arc A222 (166.5402, 21.3487) -> (166.2862, 21.6027) centre (166.2862, 21.3487) ccw
  line L337 (166.2862, 7.6073) -> (152.7988, 7.6073)
  line L338 (166.5402, 7.6073) -> (152.5448, 21.6027) construction
  line L339 (152.5448, 7.6073) -> (166.5402, 21.6027) construction
  line L340 (166.5402, 21.3487) -> (166.5402, 7.8613)
  arc A223 (166.2862, 7.6073) -> (166.5402, 7.8613) centre (166.2862, 7.8613) ccw
  arc A224 (155.1813, 2.5527) -> (154.9273, 2.2987) centre (155.1813, 2.2987) ccw
  line L341 (154.9273, -11.1887) -> (154.9273, 2.2987)
  arc A225 (154.9273, -11.1887) -> (155.1813, -11.4427) centre (155.1813, -11.1887) ccw
  line L342 (155.1813, 2.5527) -> (168.6687, 2.5527)
  arc A226 (168.9227, 2.2987) -> (168.6687, 2.5527) centre (168.6687, 2.2987) ccw
  line L343 (168.6687, -11.4427) -> (155.1813, -11.4427)
  line L344 (168.9227, -11.4427) -> (154.9273, 2.5527) construction
  line L345 (154.9273, -11.4427) -> (168.9227, 2.5527) construction
  line L346 (168.9227, 2.2987) -> (168.9227, -11.1887)
  arc A227 (168.6687, -11.4427) -> (168.9227, -11.1887) centre (168.6687, -11.1887) ccw
  arc A228 (116.5352, 40.3987) -> (116.2812, 40.6527) centre (116.2812, 40.3987) ccw
  line L347 (116.5352, 40.3987) -> (116.5352, 26.9113)
  arc A229 (116.2812, 26.6573) -> (116.5352, 26.9113) centre (116.2812, 26.9113) ccw
  line L348 (116.2812, 26.6573) -> (102.7938, 26.6573)
  line L349 (102.7938, 40.6527) -> (116.2812, 40.6527)
  line L350 (116.5352, 26.6573) -> (102.5398, 40.6527) construction
  line L351 (102.5398, 26.6573) -> (116.5352, 40.6527) construction
  arc A230 (102.7938, 40.6527) -> (102.5398, 40.3987) centre (102.7938, 40.3987) ccw
  line L352 (102.5398, 26.9113) -> (102.5398, 40.3987)
  arc A231 (102.5398, 26.9113) -> (102.7938, 26.6573) centre (102.7938, 26.9113) ccw
  arc A232 (97.4852, 40.3987) -> (97.2312, 40.6527) centre (97.2312, 40.3987) ccw
  line L353 (97.4852, 40.3987) -> (97.4852, 26.9113)
  arc A233 (97.2312, 26.6573) -> (97.4852, 26.9113) centre (97.2312, 26.9113) ccw
  line L354 (97.2312, 26.6573) -> (83.7438, 26.6573)
  line L355 (83.7438, 40.6527) -> (97.2312, 40.6527)
  line L356 (97.4852, 26.6573) -> (83.4898, 40.6527) construction
  line L357 (83.4898, 26.6573) -> (97.4852, 40.6527) construction
  arc A234 (83.7438, 40.6527) -> (83.4898, 40.3987) centre (83.7438, 40.3987) ccw
  line L358 (83.4898, 26.9113) -> (83.4898, 40.3987)
  arc A235 (83.4898, 26.9113) -> (83.7438, 26.6573) centre (83.7438, 26.9113) ccw
  arc A236 (78.4352, 40.3987) -> (78.1812, 40.6527) centre (78.1812, 40.3987) ccw
  line L359 (78.4352, 40.3987) -> (78.4352, 26.9113)
  arc A237 (78.1812, 26.6573) -> (78.4352, 26.9113) centre (78.1812, 26.9113) ccw
  line L360 (78.1812, 26.6573) -> (64.6938, 26.6573)
  line L361 (64.6938, 40.6527) -> (78.1812, 40.6527)
  line L362 (78.4352, 26.6573) -> (64.4398, 40.6527) construction
  line L363 (64.4398, 26.6573) -> (78.4352, 40.6527) construction
  arc A238 (64.6938, 40.6527) -> (64.4398, 40.3987) centre (64.6938, 40.3987) ccw
  line L364 (64.4398, 26.9113) -> (64.4398, 40.3987)
  arc A239 (64.4398, 26.9113) -> (64.6938, 26.6573) centre (64.6938, 26.9113) ccw
  arc A240 (59.3852, 40.3987) -> (59.1312, 40.6527) centre (59.1312, 40.3987) ccw
  line L365 (59.3852, 40.3987) -> (59.3852, 26.9113)
  arc A241 (59.1312, 26.6573) -> (59.3852, 26.9113) centre (59.1312, 26.9113) ccw
  line L366 (59.1312, 26.6573) -> (45.6438, 26.6573)
  line L367 (45.6438, 40.6527) -> (59.1312, 40.6527)
  line L368 (59.3852, 26.6573) -> (45.3898, 40.6527) construction
  line L369 (45.3898, 26.6573) -> (59.3852, 40.6527) construction
  arc A242 (45.6438, 40.6527) -> (45.3898, 40.3987) centre (45.6438, 40.3987) ccw
  line L370 (45.3898, 26.9113) -> (45.3898, 40.3987)
  arc A243 (45.3898, 26.9113) -> (45.6438, 26.6573) centre (45.6438, 26.9113) ccw
  arc A244 (40.3352, 40.3987) -> (40.0812, 40.6527) centre (40.0812, 40.3987) ccw
  line L371 (40.3352, 40.3987) -> (40.3352, 26.9113)
  arc A245 (40.0812, 26.6573) -> (40.3352, 26.9113) centre (40.0812, 26.9113) ccw
  line L372 (40.0812, 26.6573) -> (26.5938, 26.6573)
  line L373 (26.5938, 40.6527) -> (40.0812, 40.6527)
  line L374 (40.3352, 26.6573) -> (26.3398, 40.6527) construction
  line L375 (26.3398, 26.6573) -> (40.3352, 40.6527) construction
  arc A246 (26.5938, 40.6527) -> (26.3398, 40.3987) centre (26.5938, 40.3987) ccw
  line L376 (26.3398, 26.9113) -> (26.3398, 40.3987)
  arc A247 (26.3398, 26.9113) -> (26.5938, 26.6573) centre (26.5938, 26.9113) ccw
  arc A248 (21.2852, 40.3987) -> (21.0312, 40.6527) centre (21.0312, 40.3987) ccw
  line L377 (21.2852, 40.3987) -> (21.2852, 26.9113)
  arc A249 (21.0312, 26.6573) -> (21.2852, 26.9113) centre (21.0312, 26.9113) ccw
  line L378 (21.0312, 26.6573) -> (7.5438, 26.6573)
  line L379 (7.5438, 40.6527) -> (21.0312, 40.6527)
  line L380 (21.2852, 26.6573) -> (7.2898, 40.6527) construction
  line L381 (7.2898, 26.6573) -> (21.2852, 40.6527) construction
  arc A250 (7.5438, 40.6527) -> (7.2898, 40.3987) centre (7.5438, 40.3987) ccw
  line L382 (7.2898, 26.9113) -> (7.2898, 40.3987)
  arc A251 (7.2898, 26.9113) -> (7.5438, 26.6573) centre (7.5438, 26.9113) ccw
  arc A252 (2.2352, 40.3987) -> (1.9812, 40.6527) centre (1.9812, 40.3987) ccw
  line L383 (2.2352, 40.3987) -> (2.2352, 26.9113)
  arc A253 (1.9812, 26.6573) -> (2.2352, 26.9113) centre (1.9812, 26.9113) ccw
  line L384 (1.9812, 26.6573) -> (-11.5062, 26.6573)
  line L385 (-11.5062, 40.6527) -> (1.9812, 40.6527)
  line L386 (2.2352, 26.6573) -> (-11.7602, 40.6527) construction
  line L387 (-11.7602, 26.6573) -> (2.2352, 40.6527) construction
  arc A254 (-11.5062, 40.6527) -> (-11.7602, 40.3987) centre (-11.5062, 40.3987) ccw
  line L388 (-11.7602, 26.9113) -> (-11.7602, 40.3987)
  arc A255 (-11.7602, 26.9113) -> (-11.5062, 26.6573) centre (-11.5062, 26.9113) ccw
  arc A256 (-16.8148, 40.3987) -> (-17.0688, 40.6527) centre (-17.0688, 40.3987) ccw
  line L389 (-16.8148, 40.3987) -> (-16.8148, 26.9113)
  arc A257 (-17.0688, 26.6573) -> (-16.8148, 26.9113) centre (-17.0688, 26.9113) ccw
  line L390 (-17.0688, 26.6573) -> (-30.5562, 26.6573)
  line L391 (-30.5562, 40.6527) -> (-17.0688, 40.6527)
  line L392 (-16.8148, 26.6573) -> (-30.8102, 40.6527) construction
  line L393 (-30.8102, 26.6573) -> (-16.8148, 40.6527) construction
  arc A258 (-30.5562, 40.6527) -> (-30.8102, 40.3987) centre (-30.5562, 40.3987) ccw
  line L394 (-30.8102, 26.9113) -> (-30.8102, 40.3987)
  arc A259 (-30.8102, 26.9113) -> (-30.5562, 26.6573) centre (-30.5562, 26.9113) ccw
  arc A260 (-35.8648, 40.3987) -> (-36.1188, 40.6527) centre (-36.1188, 40.3987) ccw
  line L395 (-35.8648, 40.3987) -> (-35.8648, 26.9113)
  arc A261 (-36.1188, 26.6573) -> (-35.8648, 26.9113) centre (-36.1188, 26.9113) ccw
  line L396 (-36.1188, 26.6573) -> (-49.6062, 26.6573)
  line L397 (-49.6062, 40.6527) -> (-36.1188, 40.6527)
  line L398 (-35.8648, 26.6573) -> (-49.8602, 40.6527) construction
  line L399 (-49.8602, 26.6573) -> (-35.8648, 40.6527) construction
  arc A262 (-49.6062, 40.6527) -> (-49.8602, 40.3987) centre (-49.6062, 40.3987) ccw
  line L400 (-49.8602, 26.9113) -> (-49.8602, 40.3987)
  arc A263 (-49.8602, 26.9113) -> (-49.6062, 26.6573) centre (-49.6062, 26.9113) ccw
  arc A264 (-54.9148, 40.3987) -> (-55.1688, 40.6527) centre (-55.1688, 40.3987) ccw
  line L401 (-54.9148, 40.3987) -> (-54.9148, 26.9113)
  arc A265 (-55.1688, 26.6573) -> (-54.9148, 26.9113) centre (-55.1688, 26.9113) ccw
  line L402 (-55.1688, 26.6573) -> (-68.6562, 26.6573)
  line L403 (-68.6562, 40.6527) -> (-55.1688, 40.6527)
  line L404 (-54.9148, 26.6573) -> (-68.9102, 40.6527) construction
  line L405 (-68.9102, 26.6573) -> (-54.9148, 40.6527) construction
  arc A266 (-68.6562, 40.6527) -> (-68.9102, 40.3987) centre (-68.6562, 40.3987) ccw
  line L406 (-68.9102, 26.9113) -> (-68.9102, 40.3987)
  arc A267 (-68.9102, 26.9113) -> (-68.6562, 26.6573) centre (-68.6562, 26.9113) ccw
  line L407 (183.1975, 33.655) -> (128.5875, 33.655) construction
  arc A268 (171.3052, 59.4487) -> (171.0512, 59.7027) centre (171.0512, 59.4487) ccw
  line L408 (171.3052, 59.4487) -> (171.3052, 45.9613)
  arc A269 (171.0512, 45.7073) -> (171.3052, 45.9613) centre (171.0512, 45.9613) ccw
  line L409 (157.5638, 59.7027) -> (171.0512, 59.7027)
  line L410 (171.0512, 45.7073) -> (157.5638, 45.7073)
  line L411 (171.3052, 45.7073) -> (157.3098, 59.7027) construction
  line L412 (157.3098, 45.7073) -> (171.3052, 59.7027) construction
  arc A270 (157.3098, 45.9613) -> (157.5638, 45.7073) centre (157.5638, 45.9613) ccw
  line L413 (157.3098, 45.9613) -> (157.3098, 59.4487)
  arc A271 (157.5638, 59.7027) -> (157.3098, 59.4487) centre (157.5638, 59.4487) ccw
  line L414 (147.4927, 59.4487) -> (147.4927, 45.9613)
  arc A272 (147.2387, 45.7073) -> (147.4927, 45.9613) centre (147.2387, 45.9613) ccw
  arc A273 (147.4927, 59.4487) -> (147.2387, 59.7027) centre (147.2387, 59.4487) ccw
  line L415 (133.7513, 59.7027) -> (147.2387, 59.7027)
  line L416 (147.2387, 45.7073) -> (133.7513, 45.7073)
  line L417 (147.4927, 45.7073) -> (133.4973, 59.7027) construction
  line L418 (133.4973, 45.9613) -> (133.4973, 59.4487)
  arc A274 (133.4973, 45.9613) -> (133.7513, 45.7073) centre (133.7513, 45.9613) ccw
  arc A275 (133.7513, 59.7027) -> (133.4973, 59.4487) centre (133.7513, 59.4487) ccw
  line L419 (133.4973, 45.7073) -> (147.4927, 59.7027) construction
  line L420 (123.6802, 59.4487) -> (123.6802, 45.9613)
  arc A276 (123.4262, 45.7073) -> (123.6802, 45.9613) centre (123.4262, 45.9613) ccw
  arc A277 (123.6802, 59.4487) -> (123.4262, 59.7027) centre (123.4262, 59.4487) ccw
  line L421 (109.9388, 59.7027) -> (123.4262, 59.7027)
  line L422 (123.4262, 45.7073) -> (109.9388, 45.7073)
  line L423 (123.6802, 45.7073) -> (109.6848, 59.7027) construction
  line L424 (109.6848, 45.9613) -> (109.6848, 59.4487)
  arc A278 (109.6848, 45.9613) -> (109.9388, 45.7073) centre (109.9388, 45.9613) ccw
  arc A279 (109.9388, 59.7027) -> (109.6848, 59.4487) centre (109.9388, 59.4487) ccw
  line L425 (109.6848, 45.7073) -> (123.6802, 59.7027) construction
  line L426 (99.8677, 59.4487) -> (99.8677, 45.9613)
  arc A280 (99.6137, 45.7073) -> (99.8677, 45.9613) centre (99.6137, 45.9613) ccw
  arc A281 (99.8677, 59.4487) -> (99.6137, 59.7027) centre (99.6137, 59.4487) ccw
  line L427 (86.1263, 59.7027) -> (99.6137, 59.7027)
  line L428 (99.6137, 45.7073) -> (86.1263, 45.7073)
  line L429 (99.8677, 45.7073) -> (85.8723, 59.7027) construction
  line L430 (85.8723, 45.9613) -> (85.8723, 59.4487)